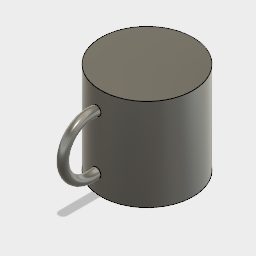
444 (Autodesk Fusion 360 design; units mm, degrees)
Autodesk Fusion 360 part; units mm, degrees
cylinder "圆柱体基本要素1" add diameter 20 height 20 placed x (1, 0, 0) y (0, 0, -1) z (0, 1, 0) at (0, 0, 0) makes body 1
cylinder "圆柱体基本要素2" add diameter 18 height 20 placed x (1, 0, 0) y (0, 0, -1) z (0, 1, 0) at (25, 0, 0) separate body makes body 2
torus "圆环体基本要素1" add centre line diameter 18 section diameter 2 placed x (-1, 0, 0) y (0, 0, 1) z (0, 1, 0) at (-25, 20, 0) separate body makes body 3
move_body "MoveFace1" bodies 3 to x (0, 1, 0) y (-1, 0, 0) z (0, 0, 1) at (15.3478, 34.8763, 24.9299) on bodies 3
delete_face "删除面1" 1 faces at (-4.9942, 8.6403, 34.7925) on bodies 3
torus "圆环体基本要素2" add centre line diameter 12 section diameter 2 placed x (1, 0, 0) y (0, 0, -1) z (0, 1, 0) at (-25, 0, 0) separate body makes body 4
torus "圆环体基本要素3" add centre line diameter 12 section diameter 2 placed x (1, 0, 0) y (0, 0, -1) z (0, 1, 0) at (-25, 0, 15) separate body makes body 5
delete_face "删除面2" 1 faces at (-30.5319, -0.342, 19.1902) on bodies 5
move_body "MoveFace2" bodies 4 to x (0, 1, 0) y (-1, 0, 0) z (0, 0, 1) at (-1.0264, 34.8586, 11.2578) on bodies 4
combine "合并1" operation add target body 4 tool bodies 1
move_body "对齐1" bodies 2 to x (1, 0, 0) y (0, 1, 0) z (0, 0, 1) at (-25, 0, 0)
move_face "偏移面2" offset -2 1 faces at (-5.1676, 20, -0.3267) on bodies 2
combine "合并3" operation cut target body 4 tool bodies 2
